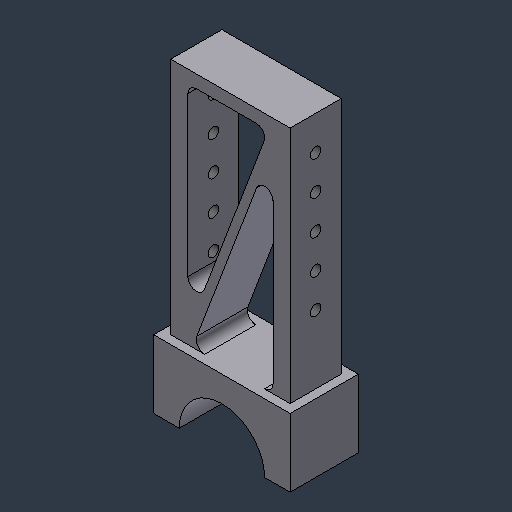
# Autodesk Inventor part: BLOCK,BEARING,ARM,ELEVATOR
Saved by Autodesk Inventor 2024.3 (Build 283343000, 343)
## iProperties
Category: _
Manager: _
ILogicPurgeVersion: 0.0.0.0
OnSaveVersion: 3.5.0.0
OnSaveAssembly: COREAutomationManager
Created: 2025-03-04
Part Number: BLOCK,BEARING,ARM,ELEVATOR
Checked By: 00
Engr Approved By: _
User Status: Work In Process
Material: Aluminum, 7075-T6
Description: STANDARD (mm)
Document SubType Name: Modeling
Mfg Approved By: John.Thibert
Designer: John.Thibert
Manufacturer: Standard
Standards Organization: Custom
Mass: 148.03 g
Surface Area: 203.938 cm^2
Volume: 52.6796 cm^3
Density: 2.81 g/cm^3
Appearance: Metal-AL-6061 (Flat)
CN_MASS: 0.15
CN_SERVICEABLE: _
FIRST_DESCRIPTION: _
SECOND_DESCRIPTION: _
THIRD_DESCRIPTION: _
ModelCat: Uncategorized
MaterialName: Aluminum, 7075-T6
Subject: _
Author: John.Thibert
Keywords: -
Revision Number: A
Autodesk Inventor part; units mm, degrees
ref_plane "YZ Plane" through (0, 0, 0) normal (1, 0, 0) x (0, 1, 0)
ref_plane "XZ Plane" through (0, 0, 0) normal (0, 1, 0) x (-1, 0, 0)
ref_plane "XY Plane" through (0, 0, 0) normal (0, 0, 1) x (1, 0, 0)
sketch "Sketch2" plane through (0, 0, 0) normal (0, 0, 1) x (1, 0, 0)
  line L0 (22.225, 0) -> (22.225, 88.9)
  line L1 (22.225, 88.9) -> (-22.225, 88.9)
  line L2 (-22.225, 88.9) -> (-22.225, 0)
  line L3 (22.225, 0) -> (25.4, 0)
  line L4 (25.4, 0) -> (25.4, -25.4)
  arc A0 (-25.4, -25.4) -> (25.4, -25.4) centre (0, -25.4) ccw
  line L5 (-25.4, -25.4) -> (-25.4, 0)
  line L6 (-25.4, 0) -> (-22.225, 0)
  line L7 (0, 116.84) -> (0, -78.74) construction
  line L8 (-35.56, 0) -> (35.56, 0) construction
  line L9 (-15.875, 84.1375) -> (15.875, 84.1375)
  line L10 (15.875, 84.1375) -> (15.875, 0)
  line L11 (15.875, 0) -> (-15.875, 0)
  line L12 (-15.875, 0) -> (-15.875, 84.1375)
  line L13 (-15.875, 84.1375) -> (15.875, 0) construction
  line L14 (15.875, 84.1375) -> (-15.875, 0) construction
  line L15 (15.875, 79.6411) -> (-14.1782, 0)
  line L16 (14.1782, 84.1375) -> (-15.875, 4.4964)
  point P0 (0, 0)
  point P1 (0, 88.9)
  point P2 (0, 42.0688)
  dimension "d0" = 44.45
  dimension "d1" = 88.9
  dimension "d2" = 25.4
  dimension "d3" = 25.4
  dimension "d6" = 6.35
  dimension "d7" = 4.7625
  dimension "d8" = 1.5875
  constraints: 30 end point, 7 point on line, 5 perpendicular, 4 parallel, 3 midpoint, 2 collinear, 2 equal length, 2 horizontal, 2 point on circle, 2 tangent, 2 vertical, 1 centre point
  measures "d0" distance of L0.end L1.end
  measures "d1" distance of L1.end L2.end
  measures "d2" distance of L5.start L5.end
  measures "d3" radius of A0
  measures "d6" distance between parallel lines of L0 L10
  measures "d7" distance between parallel lines of L1 L9
  measures "d8" distance between parallel lines of L14 L16
extrude "Extrusion1" add sketch "Sketch2" along normal mid plane 25.4 contours L3 L4 A0 L5 L6 L2 L1 L0 | L9 L10 L15 L11 L12 L16
sketch "Sketch4" plane through (0, 0, 12.7) normal (0, 0, 1) x (1, 0, 0)
  arc A0 (-25.4, -25.4) -> (25.4, -25.4) centre (0, -25.4) ccw construction
  point P0 (0, 0)
  constraints: 1 coincident
hole "Hole1" at (0, -25.4, 12.7) direction (0, 0, -1) diameter 31.75 end through all
fillet "Fillet1" radius 3.175 6 edges at (14.1782, 84.1375, 0) (-15.875, 84.1375, 0) (-15.875, 4.4964, 0) (-14.1782, 0, 0) (15.875, 79.6411, 0) (15.875, 0, 0)
sketch "Sketch5" plane through (-22.225, 0, -12.7) normal (-1, 0, 0) x (0, 0, 1)
  line L0 (0, 88.9) -> (25.4, 88.9) construction
  line L1 (12.7, 88.9) -> (12.7, 0) construction
  line L2 (12.7, 0) -> (25.4, 0) construction
  line L3 (12.7, 116.84) -> (12.7, -78.74) construction
  line L4 (0, 0) -> (25.4, 0) construction
  point P0 (12.7, 25.4)
  point P1 (12.7, 38.1)
  point P2 (12.7, 50.8)
  point P3 (12.7, 63.5)
  point P4 (12.7, 76.2)
  dimension "d21" = 12.7
  dimension "d37" = 25.4
  constraints: 2 end point, 2 point on line, 1 collinear, 1 midpoint, 1 vertical, 4 other
  measures "d21" distance of point (12.7, 25.4) point (12.7, 38.1)
  measures "d37" distance from line of L4 point (12.7, 25.4)
hole "Hole2" at (-22.225, 25.4, 0) at (-22.225, 38.1, 0) at (-22.225, 50.8, 0) at (-22.225, 63.5, 0) at (-22.225, 76.2, 0) direction (1, 0, 0) diameter 3.9624 depth 13.6144 tip angle 118 thread size "10-32 UNF" class "2B" standard "ANSI Unified Screw Threads"
mirror "Mirror1" about plane through (0, 0, 0) normal (1, 0, 0) of "Hole2"
sketch "Sketch6" plane through (0, 0, 0) normal (1, 0, 0) x (0, 1, 0)
  line L0 (0, 12.7) -> (-50.8, 12.7)
  line L1 (-50.8, 12.7) -> (-50.8, -12.7)
  line L2 (-50.8, -12.7) -> (0, -12.7)
  line L3 (0, -12.7) -> (0, 12.7)
  line L4 (-50.8, -12.7) -> (-50.8, 12.7) construction
  line L5 (0, 9.525) -> (88.9, 9.525)
  line L6 (88.9, 9.525) -> (88.9, -9.525)
  line L7 (88.9, -9.525) -> (0, -9.525)
  line L8 (0, -9.525) -> (0, 9.525)
  line L9 (88.9, -12.7) -> (88.9, 12.7) construction
  line L10 (-25.4, -12.7) -> (-25.4, 12.7) projected
  point P0 (0, 0)
  point P1 (0, 0)
  point P2 (0, -9.525)
  dimension "d33" = 25.4
  dimension "d34" = 19.05
  constraints: 16 end point, 4 parallel, 2 collinear, 2 horizontal, 2 midpoint, 2 perpendicular, 1 coincident
  measures "d33" distance of L0.end L1.end
  measures "d34" distance of L7.end L5.start
extrude "Extrusion2" cut sketch "Sketch6" along normal through all both and the other way through all contours L3 L2 L10 L0 | L5 L6 L7 L3 keep common part
sketch "Sketch7" plane through (-25.4, -25.4, 12.7) normal (0, -1, 0) x (1, 0, 0)
  line L0 (4.7625, -19.05) -> (46.0375, -19.05) construction
  line L1 (46.0375, -19.05) -> (46.0375, -6.35) construction
  line L2 (46.0375, -6.35) -> (4.7625, -6.35) construction
  line L3 (4.7625, -6.35) -> (4.7625, -19.05) construction
  line L4 (4.7625, -19.05) -> (46.0375, -6.35) construction
  line L5 (46.0375, -19.05) -> (4.7625, -6.35) construction
  point P0 (25.4, -12.7)
  point P1 (25.4, -12.7)
  dimension "d39" = 12.7
  dimension "d40" = 41.275
  constraints: 12 end point, 5 coincident, 2 midpoint, 2 parallel, 1 horizontal, 1 perpendicular
  measures "d39" distance of L0.end L1.end
  measures "d40" distance of L0.start L0.end
hole "Hole3" at (20.6375, -25.4, 6.35) at (20.6375, -25.4, -6.35) at (-20.6375, -25.4, 6.35) at (-20.6375, -25.4, -6.35) direction (0, 1, 0) diameter 3.9624 depth 13.6144 tip angle 118 thread size "10-32 UNF" class "2B" standard "ANSI Unified Screw Threads"
body "Solid1"
